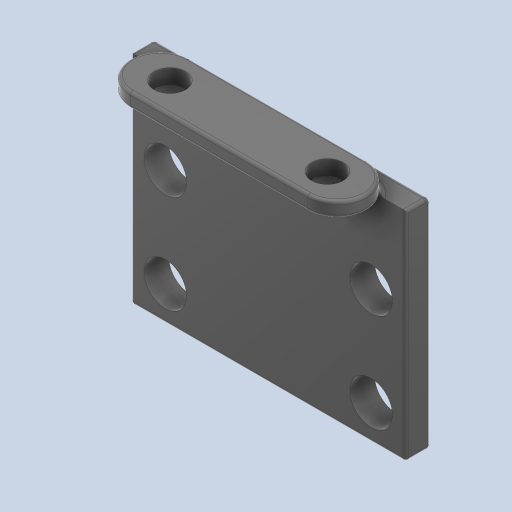
# Autodesk Inventor part: distance_sensor_hold
Saved by Autodesk Inventor 2023 (Build 270158000, 158)
## iProperties
Created: 2021-02-23
Part Number: distance_sensor_hold
Material: Generic
Document SubType Name: Modeling
Designer: JojoS
Density: 1 g/cm^3
Appearance: Default
Author: JojoS
Autodesk Inventor part; units mm, degrees
ref_plane "YZ Plane" through (0, 0, 0) normal (1, 0, 0) x (0, 1, 0)
ref_plane "XZ Plane" through (0, 0, 0) normal (0, 1, 0) x (-1, 0, 0)
ref_plane "XY Plane" through (0, 0, 0) normal (0, 0, 1) x (1, 0, 0)
sketch "Sketch1" plane through (0, 0, 0) normal (0, 0, 1) x (1, 0, 0)
  line L0 (0, 0) -> (27.9, 0)
  line L1 (27.9, 0) -> (27.9, -22.1)
  line L2 (27.9, -22.1) -> (0, -22.1)
  line L3 (0, -22.1) -> (0, 0)
  dimension "d0" = 27.9
  dimension "d1" = 22.1
  constraints: 8 end point, 2 parallel, 1 horizontal, 1 perpendicular
  measures "d0" distance of L1.end L2.end
  measures "d1" distance of L0.end L1.end
extrude "Extrusion1" add sketch "Sketch1" along normal blind 2.5
sketch "Sketch2" plane through (0, 0, 0) normal (0, 1, 0) x (1, 0, 0)
  line L0 (1.95, -4.5) -> (25.95, -4.5) construction
  line L1 (4.95, -7.5) -> (22.95, -7.5)
  line L2 (22.95, -1.5) -> (4.95, -1.5)
  arc A0 (4.95, -1.5) -> (4.95, -7.5) centre (4.95, -4.5) ccw
  arc A1 (22.95, -7.5) -> (22.95, -1.5) centre (22.95, -4.5) ccw
  line L3 (27.9, 0) -> (27.9, -2.5) projected
  line L4 (0, 0) -> (0, -2.5) projected
  line L5 (27.9, -2.5) -> (0, -2.5) projected
  circle A2 centre (5.95, -4.5) radius 1.6
  circle A3 centre (21.95, -4.5) radius 1.6
  line L6 (4.752, -3.4394) -> (4.752, -5.5606)
  line L7 (0, 0) -> (27.9, 0) projected
  line L8 (13.95, 0) -> (13.95, -7.0714)
  point P0 (13.95, -4.5)
  dimension "d4" = 6
  dimension "d5" = 24
  dimension "d8" = 1
  dimension "d9" = 3.2
  dimension "d10" = 3.2
  dimension "d11" = 16
  dimension "d12" = 8
  constraints: 12 end point, 8 point on circle, 5 point on line, 4 centre point, 4 tangent, 2 midpoint, 2 vertical, 1 horizontal, 1 parallel
  measures "d4" diameter of A1
  measures "d5" distance of L0.start L0.end
  measures "d8" distance between parallel lines of L5 L2
  measures "d9" diameter of A2
  measures "d10" diameter of A3
  measures "d11" distance of A3.centre A2.centre
  measures "d12" distance of point (13.95, -4.5) A2.centre
extrude "Extrusion2" add sketch "Sketch2" along normal blind 1.5 contours A0 L5 A1 L1 | A0 L2 L8 L5 | L5 L8 L2 A1
fillet "Fillet1" radius 0.3 4 edges at (1.95, 1.5, 4.5) (13.95, 1.5, 7.5) (25.95, 1.5, 4.5) (13.95, 1.5, 1.5)
fillet "Fillet2" radius 0.5 3 edges at (13.95, 0, 1.5) (13.95, 0, 0) (13.95, 0, 2.5)
fillet "Fillet3" radius 0.3 3 edges at (25.5481, 0, 6) (2.3519, 0, 6) (13.95, 0, 7.5)
sketch "Sketch3" plane through (0, 0, 0) normal (0, 0, -1) x (-1, 0, 0)
  circle A0 centre (-24.4, -18.6) radius 2.15
  line L0 (-27.9, -22.1) -> (-27.9, -0.5) projected
  line L1 (0, -22.1) -> (-27.9, -22.1) projected
  line L2 (-13.95, -22.1) -> (-13.95, -20.8715)
  circle A1 centre (-24.4, -8.6) radius 2.15
  line L3 (0, 0) -> (-27.9, 0) projected
  circle A2 centre (-3.5, -18.6) radius 2.15
  circle A3 centre (-3.5, -8.6) radius 2.15
  point P0 (-27.9, -11.3)
  point P1 (0, -11.3)
  dimension "d19" = 4.3
  dimension "d23" = 3.5
  dimension "d28" = 8.6
  dimension "d29" = 3.5
  dimension "d30" = 4.3
  dimension "d31" = 3.5
  constraints: 4 centre point, 3 symmetric about line, 2 end point, 2 midpoint, 1 vertical, 2 other
  measures "d19" diameter of A0
  measures "d23" distance from line of L0 A0.centre
  measures "d28" distance from line of L3 A1.centre
  measures "d29" horizontal distance of point (-27.9, -11.3) A1.centre
  measures "d30" diameter of A1
  measures "d31" distance from line of L1 A0.centre
fillet "Fillet4" radius 0.3 12 edges at (27.9, -0.1464, 0.1464) (27.9, 0, 1.5) (27.9, -11.3, 0) (27.9, -11.05, 2.5) (13.95, -22.1, 0) (27.9, -22.1, 1.25) (13.95, -22.1, 2.5) (0, -22.1, 1.25) (0, -0.1464, 0.1464) (0, 0, 1.5) (0, -11.3, 0) (0, -11.05, 2.5)
extrude "Extrusion3" cut sketch "Sketch3" against normal blind 5
body "Solid1"
